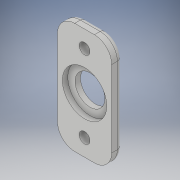
# Autodesk Inventor part: sides
Saved by Autodesk Inventor 2019 (Build 230136000, 136)
## iProperties
Created: 2018-08-03
Part Number: sides
Material: Generic
Document SubType Name: Modeling
Designer: Brian
Density: 1 g/cm^3
Appearance: Default
Author: Brian
Autodesk Inventor part; units mm, degrees
ref_plane "YZ Plane" through (0, 0, 0) normal (1, 0, 0) x (0, 1, 0)
ref_plane "XZ Plane" through (0, 0, 0) normal (0, 1, 0) x (-1, 0, 0)
ref_plane "XY Plane" through (0, 0, 0) normal (0, 0, 1) x (1, 0, 0)
sketch "Sketch1" plane through (0, 0, 0) normal (0, 0, 1) x (1, 0, 0)
  line L0 (0, 0) -> (20, 0)
  line L1 (20, 0) -> (20, 41)
  line L2 (20, 41) -> (0, 41)
  line L3 (0, 41) -> (0, 0)
  dimension "d0" = 20
  dimension "d1" = 41
  constraints: 8 end point, 2 parallel, 1 horizontal, 1 perpendicular
  measures "d0" distance of L2.end L1.end
  measures "d1" distance of L0.end L1.end
extrude "Extrusion1" add sketch "Sketch1" along normal blind 4
sketch "Sketch2" plane through (0, 0, 4) normal (0, 0, 1) x (1, 0, 0)
  line L0 (20, 0) -> (20, 41) projected
  line L1 (20, 41) -> (0, 41) projected
  point P0 (0, 0)
  point P1 (10, 20.5)
  dimension "d11" = 10
  dimension "d12" = 20.5
  measures "d11" distance from line of L0 point (10, 20.5)
  measures "d12" distance from line of L1 point (10, 20.5)
hole "Hole1" at (10, 20.5, 4) direction (0, 0, -1) diameter 11 end through all counterbore diameter 16.4 counterbore depth 2
sketch "Sketch3" plane through (0, 0, 4) normal (0, 0, 1) x (1, 0, 0)
  line L0 (20, 0) -> (20, 41) projected
  line L1 (20, 41) -> (0, 41) projected
  point P0 (0, 0)
  point P1 (10, 34.75)
  dimension "d20" = 10
  dimension "d21" = 6.25
  measures "d20" distance from line of L0 point (10, 34.75)
  measures "d21" distance from line of L1 point (10, 34.75)
hole "Hole2" at (10, 34.75, 4) direction (0, 0, -1) diameter 4 end through all
sketch "Sketch4" plane through (0, 0, 4) normal (0, 0, 1) x (1, 0, 0)
  line L0 (20, 0) -> (20, 41) projected
  line L1 (0, 0) -> (20, 0) projected
  point P0 (10, 6.25)
  dimension "d29" = 10
  dimension "d30" = 6.25
  measures "d29" distance from line of L0 point (10, 6.25)
  measures "d30" distance from line of L1 point (10, 6.25)
hole "Hole3" at (10, 6.25, 4) direction (0, 0, -1) diameter 4 end through all
fillet "Fillet1" radius 6.35 1 edges at (20, 41, 2)
fillet "Fillet2" radius 6.35 1 edges at (0, 41, 2)
fillet "Fillet3" radius 6.35 1 edges at (20, 0, 2)
fillet "Fillet4" radius 6.35 1 edges at (0, 0, 2)
fillet "Fillet5" radius 1.905 8 edges at (10, 41, 0) (1.8599, 39.1401, 0) (0, 20.5, 0) (1.8599, 1.8599, 0) (10, 0, 0) (18.1401, 1.8599, 0) (20, 20.5, 0) (18.1401, 39.1401, 0)
body "Solid1"
